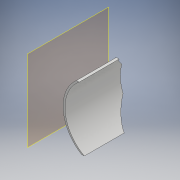
# Autodesk Inventor part: 12mm_radius_mold_with_crystal_skull
Saved by Autodesk Inventor 2018 (Build 220112000, 112)
## iProperties
Created: 2018-06-11
Part Number: 12mm_radius_mold_with_crystal_skull
Material: Generic
Document SubType Name: Modeling
Designer: McCormick Lab
Density: 1 g/cm^3
Appearance: Default
Author: McCormick Lab
Autodesk Inventor part; units mm, degrees
ref_plane "YZ Plane" through (0, 0, 0) normal (1, 0, 0) x (0, 1, 0)
ref_plane "XZ Plane" through (0, 0, 0) normal (0, 1, 0) x (-1, 0, 0)
ref_plane "XY Plane" through (0, 0, 0) normal (0, 0, 1) x (1, 0, 0)
sketch "Sketch1" plane through (0, 0, 0) normal (0, 1, 0) x (-1, 0, 0)
  arc A0 (0, -6) -> (0, 6) centre (0, 0) ccw
  line L0 (0, 6) -> (0, -6)
  dimension "d0" = 12
  constraints: 2 end point, 2 point on circle, 1 centre point, 1 coincident, 1 vertical
  measures "d0" diameter of A0
extrude "Extrusion1" add sketch "Sketch1" along normal blind 12
ref_plane "Work Plane1" through (-10, 0, 6) normal (1, 0, 0) x (0, 0, -1)
sketch "Sketch2" plane through (-10, 0, 6) normal (1, 0, 0) x (0, 0, -1)
  line L0 (1.2731, 8.0057) -> (1.2731, 1.5057)
  line L1 (1.2731, 1.5057) -> (11.2731, 1.5057)
  line L2 (11.2731, 1.5057) -> (11.2731, 8)
  line L3 (8.2731, 10.5) -> (4.2731, 10.5)
  line L4 (8.2731, 10.5) -> (11.2731, 8)
  line L5 (4.2731, 10.5) -> (1.2731, 8.0057)
  point P0 (6, 0)
  dimension "d9" = 10
  dimension "d10" = 6.5
  dimension "d12" = 4
  dimension "d14" = 3
  dimension "d15" = 3
  constraints: 12 end point, 1 horizontal, 1 parallel
  measures "d9" distance of L1.end L0.end
  measures "d10" distance of L0.end L0.start
  measures "d12" distance of L3.start L3.end
  measures "d14" horizontal distance of L0.end L3.end
  measures "d15" horizontal distance of L3.start L2.end
extrude "Extrusion2" add sketch "Sketch2" along normal blind 10
sketch "Sketch3" plane through (0, 0, 0) normal (0, 1, 0) x (-1, 0, 0)
  arc A0 (0, -6) -> (0, 6) centre (0, 0) ccw projected
  arc A1 (0, -6) -> (0, 6) centre (0, 0) ccw
  line L0 (0, 6) -> (0, -6) projected
  line L1 (0, -6) -> (0, 6)
  constraints: 2 end point, 2 point on circle, 1 centre point, 1 collinear
extrude "Extrusion3" cut sketch "Sketch3" along normal through all both and the other way through all
sketch "Sketch4" plane through (0, 0, 0) normal (0, 1, 0) x (-1, 0, 0)
  line L0 (2.8626, -5.2731) -> (3.3126, -5.2731)
  line L1 (3.6955, 4.7269) -> (4.1455, 4.7269)
  arc A0 (3.3126, -5.2731) -> (4.1455, 4.7269) centre (0.1386, 0.0259) ccw
  arc A1 (2.8626, -5.2731) -> (3.6955, 4.7269) centre (7.9551, -0.6626) ccw
  point P0 (0, 0)
  dimension "d20" = 0.45
  dimension "d21" = 0.45
  constraints: 4 end point, 4 point on circle, 2 centre point
  measures "d20" distance of L0.start L0.end
  measures "d21" distance of L1.end L1.start
extrude "Extrusion4" cut sketch "Sketch4" along normal through all
body "Solid1"
